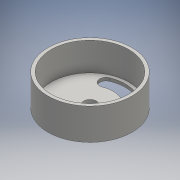
# Autodesk Inventor part: principal
Saved by Autodesk Inventor 2016 (Build 200138000, 138)
## iProperties
Created: 2016-04-19
Part Number: principal
Material: Generic
Document SubType Name: Modeling
Designer: Administrator
Density: 1 g/cm^3
Appearance: Default
Author: Administrator
Autodesk Inventor part; units mm, degrees
ref_plane "YZ Plane" through (0, 0, 0) normal (1, 0, 0) x (0, 1, 0)
ref_plane "XZ Plane" through (0, 0, 0) normal (0, 1, 0) x (-1, 0, 0)
ref_plane "XY Plane" through (0, 0, 0) normal (0, 0, 1) x (1, 0, 0)
sketch "Sketch1" plane through (0, 0, 0) normal (0, 0, 1) x (1, 0, 0)
  circle A0 centre (0, 0) radius 20
  dimension "d0" = 40
  constraints: 1 centre point, 1 coincident
  measures "d0" diameter of A0
extrude "Extrusion1" add sketch "Sketch1" along normal blind 15
shell "Shell1" thickness 1.5 removed faces 1 at (-2.364, 6.2334, 15)
sketch "Sketch2" plane through (0, 0, 1.5) normal (0, 0, 1) x (1, 0, 0)
  circle A0 centre (0, 0) radius 3
  arc A1 (5.3174, 12.9509) -> (-5.3174, 12.9509) centre (0, 0) ccw construction
  arc A2 (6.4569, 15.726) -> (-6.4569, 15.726) centre (0, 0) ccw
  arc A3 (4.178, 10.1757) -> (-4.178, 10.1757) centre (0, 0) ccw
  arc A4 (4.178, 10.1757) -> (6.4569, 15.726) centre (5.3174, 12.9509) ccw
  arc A5 (-6.4569, 15.726) -> (-4.178, 10.1757) centre (-5.3174, 12.9509) ccw
  line L0 (0, -30.6) -> (0, 43.6) projected
  dimension "d4" = 6
  dimension "d5" = 6
  dimension "d6" = 14
  constraints: 10 point on circle, 6 centre point, 4 tangent, 1 coincident, 1 symmetric about line
  measures "d4" diameter of A0
  measures "d5" diameter of A4
  measures "d6" radius of A1
extrude "Extrusion2" cut sketch "Sketch2" against normal through all
body "Solid1"
